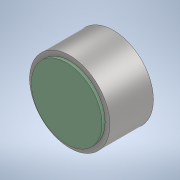
# Autodesk Inventor part: Mic_Unidirectional
Saved by Autodesk Inventor 2022 (Build 260153000, 153)
## iProperties
Created: 2022-12-26
Part Number: Mic_Unidirectional
Material: Generic
Document SubType Name: Modeling
Designer: karpova
Density: 1 g/cm^3
Appearance: Stainless - Brushed
Author: karpova
Autodesk Inventor part; units mm, degrees
ref_plane "YZ Plane" through (0, 0, 0) normal (1, 0, 0) x (0, 1, 0)
ref_plane "XZ Plane" through (0, 0, 0) normal (0, 1, 0) x (-1, 0, 0)
ref_plane "XY Plane" through (0, 0, 0) normal (0, 0, 1) x (1, 0, 0)
sketch "Sketch1" plane through (0, 0, 0) normal (0, 0, 1) x (1, 0, 0)
  circle A0 centre (0, 0) radius 4
  dimension "d0" = 8
  constraints: 1 centre point, 1 coincident
  measures "d0" diameter of A0
extrude "Extrusion1" add sketch "Sketch1" along normal blind 4.35
sketch "Sketch2" plane through (0, 0, 4.35) normal (0, 0, 1) x (1, 0, 0)
  circle A0 centre (0, 0) radius 3.525
  circle A1 centre (0, 0) radius 4 projected
  dimension "d16" = 7.05
  constraints: 1 centre point, 1 coincident
  measures "d16" diameter of A0
extrude "Extrusion2" add sketch "Sketch2" along normal blind 0.3 contours A0
sketch "Sketch3" plane through (0, 0, 0) normal (0, 0, -1) x (-1, 0, 0)
  circle A0 centre (0, 0) radius 3.15
  circle A1 centre (0, 0) radius 4 projected
  dimension "d17" = 6.3
  constraints: 1 centre point, 1 coincident
  measures "d17" diameter of A0
extrude "Extrusion3" cut sketch "Sketch3" against normal blind 0.3 contours A0
sketch "Sketch4" plane through (0, 0, 0.3) normal (0, 0, -1) x (-1, 0, 0)
  arc A0 (2, 0.7181) -> (-2, 0.7181) centre (0, 0) ccw
  line L0 (2, 0.7181) -> (2, 0.25)
  line L1 (2, 0.25) -> (0, 0.25)
  line L2 (-2, 0.25) -> (-2, 0.7181)
  circle A1 centre (0, 0) radius 3.525 construction
  circle A2 centre (0, 0) radius 3.15 construction
  line L3 (0, 0) -> (0, 3.15) construction
  line L4 (0, 0.25) -> (-2, 0.25)
  line L5 (0, 0) -> (3.15, 0) construction
  arc A3 (-2, -0.7181) -> (2, -0.7181) centre (0, 0) ccw
  line L6 (2, -0.7181) -> (2, -0.25)
  line L7 (2, -0.25) -> (0, -0.25)
  line L8 (-2, -0.25) -> (-2, -0.7181)
  line L9 (0, -0.25) -> (-2, -0.25)
  dimension "d9" = 1.4
  dimension "d10" = 2
  dimension "d12" = 0.5
  constraints: 20 end point, 6 point on circle, 5 symmetric about line, 3 horizontal, 2 centre point, 2 vertical, 1 coincident, 1 collinear, 1 parallel, 1 point on line, 1 other
  measures "d9" radial gap between concentric circles of A1 A0
  measures "d10" distance between parallel lines of L3 L0
  measures "d12" distance between parallel lines of L7 L1
extrude "Extrusion4" add sketch "Sketch4" along normal blind 0.25
fillet "Fillet1" radius 0.25 8 edges at (0, 2.125, 0.05) (2, 0.484, 0.05) (0, 0.25, 0.05) (-2, 0.484, 0.05) (0, -0.25, 0.05) (2, -0.484, 0.05) (0, -2.125, 0.05) (-2, -0.484, 0.05)
equation "\"d9\" = leadInset"
equation "\"d10\" = 0.5 * leadWidth"
equation "\"d12\" = leadSeparation"
equation "\"d13\" = leadExtrusion"
equation "\"d15\" = leadExtrusion"
equation "\"membraneInset\" = 0.25"
equation "\"backplateInset\" = membraneInset"
equation "\"backplateExtrusion\" = 0.125"
equation "\"leadInset\" = 1.4"
equation "\"leadSeparation\" = 0.5"
equation "\"leadWidth\" = 4"
equation "\"leadExtrusion\" = 2 * backplateExtrusion"
body "Solid1"
